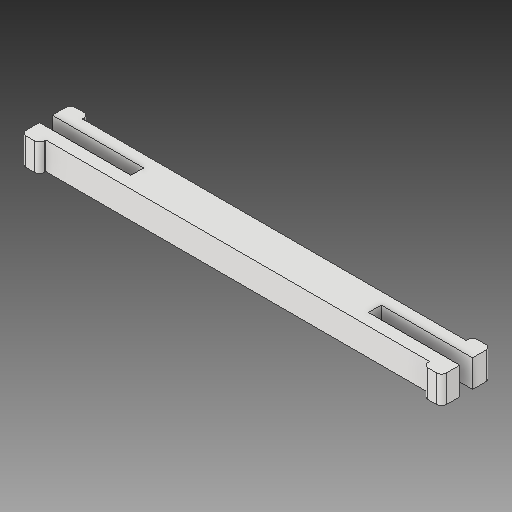
# Autodesk Inventor part: Motor Mount Slot Lock
Saved by Autodesk Inventor 2018 (Build 220112000, 112)
## iProperties
Created: 2018-01-25
Part Number: Motor Mount Slot Lock
Material: ABS Plastic
Document SubType Name: Modeling
Designer: Moochster
Density: 1.06 g/cm^3
Appearance: Smooth - White
Mass: 0.512523 g
Surface Area: 7.53991 cm^2
Volume: 0.483512 cm^3
Author: Moochster
Autodesk Inventor part; units mm, degrees
ref_plane "YZ Plane" through (0, 0, 0) normal (1, 0, 0) x (0, 1, 0)
ref_plane "XZ Plane" through (0, 0, 0) normal (0, 1, 0) x (-1, 0, 0)
ref_plane "XY Plane" through (0, 0, 0) normal (0, 0, 1) x (1, 0, 0)
sketch "Sketch1" plane through (0, 0, 0) normal (0, 1, 0) x (-1, 0, 0)
  line L0 (0, -2) -> (-21, -2)
  line L1 (-21, -2) -> (-21, -2.7)
  line L2 (0, -2) -> (0, 0) construction
  line L3 (0, 0) -> (-23, 0) construction
  line L4 (-21, -2.7) -> (-23, -2.7)
  line L5 (-23, -2.7) -> (-23, -0.7)
  line L6 (-23, -0.7) -> (-13, -0.7)
  line L7 (-13, -0.7) -> (-13, 0)
  line L8 (0, 2) -> (-21, 2)
  line L9 (-21, 2) -> (-21, 2.7)
  line L10 (-21, 2.7) -> (-23, 2.7)
  line L11 (-23, 2.7) -> (-23, 0.7)
  line L12 (-23, 0.7) -> (-13, 0.7)
  line L13 (-13, 0.7) -> (-13, 0)
  line L14 (0, -2) -> (21, -2)
  line L15 (21, -2) -> (21, -2.7)
  line L16 (21, -2.7) -> (23, -2.7)
  line L17 (23, -2.7) -> (23, -0.7)
  line L18 (23, -0.7) -> (13, -0.7)
  line L19 (13, -0.7) -> (13, 0)
  line L20 (0, 2) -> (21, 2)
  line L21 (21, 2) -> (21, 2.7)
  line L22 (21, 2.7) -> (23, 2.7)
  line L23 (23, 2.7) -> (23, 0.7)
  line L24 (23, 0.7) -> (13, 0.7)
  line L25 (13, 0.7) -> (13, 0)
  dimension "d0" = 23
  dimension "d1" = 2
  dimension "d2" = 0.7
  dimension "d3" = 10
  dimension "d4" = 0.7
  dimension "d5" = 2
  constraints: 52 end point, 17 symmetric about line, 4 perpendicular, 3 horizontal, 2 coincident, 1 point on line, 1 vertical
  measures "d0" distance from line of point (0, 0) L5
  measures "d1" distance between parallel lines of L3 L0
  measures "d2" distance between parallel lines of L3 L6
  measures "d3" distance between parallel lines of L5 L7
  measures "d4" distance between parallel lines of L0 L4
  measures "d5" distance between parallel lines of L5 L1
extrude "Extrusion1" add sketch "Sketch1" along normal blind 3
fillet "Fillet1" radius 0.5 8 edges at (21, 1.5, 2.7) (23, 1.5, 2.7) (23, 1.5, -2.7) (21, 1.5, -2.7) (-21, 1.5, 2.7) (-23, 1.5, 2.7) (-21, 1.5, -2.7) (-23, 1.5, -2.7)
body "Solid1"
